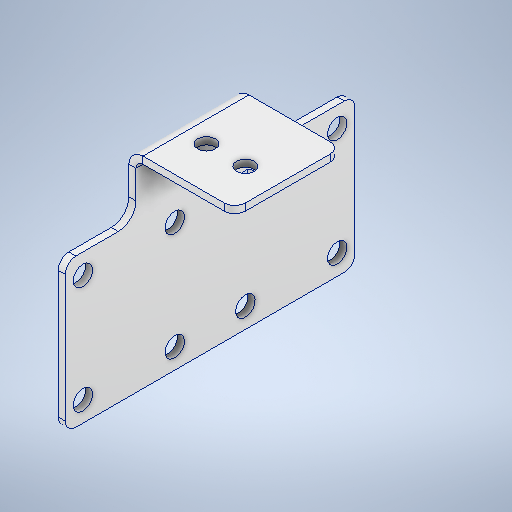
# Autodesk Inventor part: DRAGCABLE_XATTACH
Saved by Autodesk Inventor 2025.2 (Build 292293000, 293)
## iProperties
Created: 2026-03-18
Part Number: DRAGCABLE_XATTACH
Material: Aluminum 6061
Document SubType Name: Sheet Metal
Designer: composite
Density: 2.7 g/cm^3
Sheet Metal Rule: Default_mm
Appearance: Aluminum - Flat
Author: composite
Autodesk Inventor part; units mm, degrees
ref_plane "YZ Plane" through (0, 0, 0) normal (1, 0, 0) x (0, 1, 0)
ref_plane "XZ Plane" through (0, 0, 0) normal (0, 1, 0) x (-1, 0, 0)
ref_plane "XY Plane" through (0, 0, 0) normal (0, 0, 1) x (1, 0, 0)
sketch "Sketch1" plane through (0, 0, 0) normal (1, 0, 0) x (0, 1, 0)
  circle A0 centre (0, 0) radius 2.75
  line L0 (0, 0) -> (0, -2.75) construction
  line L1 (0, 0) -> (-2.75, 0) construction
  circle A1 centre (0, -26) radius 2.75
  circle A2 centre (-30.5, 0) radius 2.75
  circle A3 centre (-30.5, -26) radius 2.75
  circle A4 centre (0, -46) radius 2.75
  line L2 (0, -46) -> (0, -48.75) construction
  line L3 (0, -46) -> (-2.75, -46) construction
  circle A5 centre (0, -72) radius 2.75
  circle A6 centre (-30.5, -46) radius 2.75
  circle A7 centre (-30.5, -72) radius 2.75
  line L4 (5.75, 5) -> (-36.25, 5)
  line L5 (-36.25, 5) -> (-36.25, -77)
  line L6 (-36.25, -77) -> (5.75, -77)
  line L7 (5.75, -10) -> (5.75, 5)
  line L8 (10.75, -15) -> (20.75, -15)
  line L9 (20.75, -15) -> (20.75, -45)
  line L10 (20.75, -45) -> (10.75, -45)
  arc A8 (5.75, -10) -> (10.75, -15) centre (10.75, -10) ccw
  line L11 (5.75, -77) -> (5.75, -50)
  arc A9 (10.75, -45) -> (5.75, -50) centre (10.75, -50) ccw
  point P0 (0, -28.75)
  point P1 (-2.75, -26)
  point P2 (-30.5, -2.75)
  point P3 (-33.25, 0)
  point P4 (-30.5, -28.75)
  point P5 (-33.25, -26)
  point P6 (0, -74.75)
  point P7 (-2.75, -72)
  point P8 (-30.5, -48.75)
  point P9 (-33.25, -46)
  point P10 (-30.5, -74.75)
  point P11 (-33.25, -72)
  point P12 (5.75, -45)
  dimension "d0" = 5.5
  dimension "d3" = 26
  dimension "d6" = 30.5
  dimension "d11" = 46
  dimension "d16" = 5
  dimension "d17" = 5.75
  dimension "d18" = 5
  dimension "d19" = 5.75
  dimension "d21" = 20
  dimension "d22" = 15
  dimension "d23" = 30
  dimension "d24" = 5
  dimension "d25" = 5
  measures "d0" diameter of A0
  measures "d3" distance of L0.start A1.centre
  measures "d6" distance of L0.start A2.centre
  measures "d11" distance of point (0, 0) point (0, -46)
  measures "d16" distance from line of L4 point (0, 0)
  measures "d17" distance from line of L7 point (0, 0)
  measures "d18" distance from line of A7.centre L6
  measures "d19" distance from line of L5 A7.centre
  measures "d21" distance between parallel lines of L8 L4
  measures "d22" distance of L9.end point (5.75, -45)
  measures "d23" distance of L8.end L9.end
  measures "d24" radius of A8
  measures "d25" radius of A9
extrude "Plate1" add sketch "Sketch1" along normal blind 2
sketch "Sketch3" plane through (0, 22.75, -15) normal (0, -1, 0) x (1, 0, 0)
  line L0 (0, -30) -> (0, 0)
  line L1 (0, 0) -> (30, 0)
  line L2 (30, 0) -> (30, -30)
  line L3 (30, -30) -> (0, -30)
  constraints: 8 end point
edge flange "Flange1" height 30 angle 90 thickness 2 bend radius 2 thickness toward (0, -1, 0) relief straight relief width 2 relief depth 1 edges at (2, 20.75, -30) wall of the first edge with corners at (0, 22.75, -45) (0, 22.75, -15) (30, 22.75, -15) (30, 22.75, -45)
bend "Bend1"
corner "Corner1"
fillet "Corner Round1" radius 3 2 edges at (30, 21.75, -15) (30, 21.75, -45)
sketch "Sketch4" plane through (4, 22.75, -15) normal (0, 1, 0) x (1, 0, 0)
  circle A0 centre (6, 12) radius 2.5
  circle A1 centre (17, 12) radius 2.5
  line L0 (17, 12) -> (6, 12) construction
  line L1 (23, 0) -> (0, 0) projected
  point P0 (-4, -15)
  point P1 (11.5, 12)
  point P2 (11.5, 0)
  dimension "d37" = 5
  dimension "d38" = 5
  dimension "d39" = 11
  dimension "d40" = 12
  constraints: 2 centre point, 2 end point, 2 midpoint, 1 horizontal, 1 vertical alignment
  measures "d37" diameter of A0
  measures "d38" diameter of A1
  measures "d39" distance of L0.end L0.start
  measures "d40" distance from line of L1 L0.start
extrude "Cut1" cut sketch "Sketch4" against normal blind 2
fillet "Corner Round2" radius 3 4 edges at (1, 5.75, 5) (1, -36.25, 5) (1, 5.75, -77) (1, -36.25, -77)
equation "\"d18\" = d16"
equation "\"d37\" = d38"
equation "\"d41\" = Thickness"
equation "\"d20\" = Thickness"
equation "\"d26\" = BendReliefWidth"
equation "\"d27\" = BendReliefDepth"
equation "\"d28\" = MinimumRemnant"
equation "\"d29\" = TransitionRadius"
equation "\"d32\" = BendRadius"
equation "\"d33\" = CornerReliefSize"
equation "\"d34\" = GapSize"
equation "\"d35\" = JacobiRadiusSize"
equation "\"BendRadius\" = Thickness"
equation "\"BendReliefWidth\" = Thickness"
equation "\"BendReliefDepth\" = 0.5 * Thickness"
equation "\"CornerReliefSize\" = 4 * Thickness"
equation "\"MinimumRemnant\" = 2 * Thickness"
equation "\"TransitionRadius\" = BendRadius"
equation "\"JacobiRadiusSize\" = BendRadius"
equation "\"GapSize\" = Thickness"
equation "\"Thickness\" = 2"
body "Solid1"
